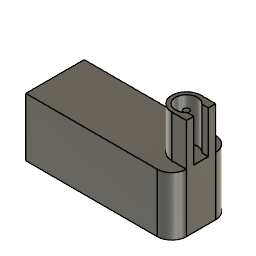
hexbug_rectangular_station_onepin (Autodesk Fusion 360 design; units mm, degrees)
Autodesk Fusion 360 part; units mm, degrees
sketch "Sketch1" plane through (0, 0, 0) normal (0, 0, 1) x (1, 0, 0)
  line L0 (0, 0) -> (-10, 0)
  line L1 (-10, 0) -> (-10, 20)
  line L2 (-10, 20) -> (0, 20)
  line L3 (0, 20) -> (0, 0)
  circle A0 centre (-5, 10) radius 5
  circle A1 centre (-5, 10) radius 3.75
  circle A2 centre (-5, 10) radius 1
  line L4 (0, 10) -> (0, 12.5)
  line L5 (0, 10) -> (0, 7.5)
  line L6 (0, 7.5) -> (0, 5)
  line L7 (0, 5) -> (-5, 5)
  line L8 (0, 7.5) -> (-2.2049, 7.5)
  line L9 (0, 12.5) -> (-2.2049, 12.5)
  line L10 (0, 12.5) -> (0, 15)
  line L11 (0, 15) -> (-5, 15)
  dimension "d1" = 20
  dimension "d2" = 10
  dimension "d3" = 7.5
  dimension "d4" = 2
  dimension "d5" = 2.5
  dimension "d6" = 2.5
  dimension "d7" = 2.5
  dimension "d8" = 2.5
  constraint horizontal L0
  constraint vertical L1
  constraint horizontal L2
  constraint vertical L3
  constraint coincident L0.start L3.end
  constraint concentric A0 A1
  constraint concentric A1 A2
  constraint midpoint L3 L4.start
  constraint parallel L3 L4
  constraint parallel L3 L5
  constraint parallel L3 L6
  constraint coincident A0 L7.end
  constraint tangent A0 L7
  constraint perpendicular L3 L7
  constraint coincident A1 L8.end
  constraint perpendicular L6 L8
  constraint coincident A1 L9.end
  constraint perpendicular L3 L9
  constraint perpendicular L9 L10
  constraint coincident A0 L11.end
  constraint tangent A0 L11
  constraint perpendicular L10 L11
  measures "d1" distance of L0.start L2.end
  measures "d2" distance of L0.start L0.end
  measures "d3" diameter of A1
  measures "d4" diameter of A2
  measures "d5" distance of L4.start L4.end
  measures "d6" distance of L4.start L5.end
  measures "d7" distance of L5.end L6.end
  measures "d8" distance of L4.end L10.end
extrude "Extrude1" add sketch "Sketch1" along normal blind 14.44 contours L3 A0 L6 L7 L8 | A0 A1 L8 L9 | L3 A0 L9 L10 L11 picked at (-1.6316, 13.0942) makes body 1
extrude "Extrude2" add sketch "Sketch1" along normal blind 14.44 separate body contours A2 makes body 2
extrude "Extrude3" add sketch "Sketch1" against normal blind 10 contours L0 L1 L3 A0 L7 | L3 A0 L6 L7 L8 | L1 L2 L3 A0 L11 | A0 A1 L8 L9 | L3 A0 L5 L8 | L3 A0 L9 L10 L11 | L3 A0 L4 L9 | A0 A1 L8 L9 | A1 | A2 bodies 1 2
extrude "Extrude4" add 1 faces at (-10, 10, -6.6667) along direction (-1, 0, 0) blind 10 on bodies 1 bodies 1
sketch "Sketch2" plane through (0, 0, 0) normal (0, 0, 1) x (-1, 0, 0)
  line L0 (5, -15) -> (0, -15)
  line L1 (0, -15) -> (0, -20)
  line L2 (0, -20) -> (20, -20)
  line L3 (20, -20) -> (20, 0)
  line L4 (20, 0) -> (0, 0)
  line L5 (0, 0) -> (0, -5)
  line L6 (0, -5) -> (5, -5)
  arc A0 (5, -15) -> (5, -5) centre (5, -10) ccw
  line L7 (10, 0) -> (20, 0)
  line L8 (20, 0) -> (20, -20)
  line L9 (20, -20) -> (10, -20)
  line L10 (10, -20) -> (10, 0)
  constraint horizontal L7
  constraint vertical L8
  constraint horizontal L9
  constraint vertical L10
  constraint coincident L2.end L3.start
  constraint midpoint L4 L7.start
extrude "Extrude5" add 1 faces at (-20, 6.6667, -3.3333) along direction (-1, 0, 0) blind 30 on bodies 1 bodies 1
fillet "Fillet1" radius 5 1 edges at (0, 0, -5) on bodies 1
fillet "Fillet2" radius 5 1 edges at (0, 20, -5) on bodies 1
extrude "Extrude6" cut 1 faces at (-4.5927, 9.5343, 14.44) along direction (0, 0, -1) blind 2 on bodies 1 bodies 1
extrude "Extrude7" add 1 faces at (-20, 13.3333, -10) along direction (0, 0, -1) blind 10 on bodies 1 bodies 1
